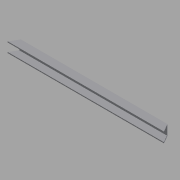
# Autodesk Inventor part: 19in c-channel-top
Saved by Autodesk Inventor 2013 (Build 170138000, 138)
## iProperties
Created: 2013-01-24
Part Number: 19in c-channel-top
Material: Generic
Document SubType Name: Modeling
Designer: Naphat
Density: 1 g/cm^3
Author: Naphat
Autodesk Inventor part; units mm, degrees
ref_plane "YZ Plane" through (0, 0, 0) normal (1, 0, 0) x (0, 1, 0)
ref_plane "XZ Plane" through (0, 0, 0) normal (0, 1, 0) x (-1, 0, 0)
ref_plane "XY Plane" through (0, 0, 0) normal (0, 0, 1) x (1, 0, 0)
sketch "Sketch1" plane through (0, 0, 0) normal (1, 0, 0) x (0, 1, 0)
  line L0 (-15.7, 12.7) -> (-12.7, 12.7)
  line L1 (-12.7, 12.7) -> (-12.7, -9.7)
  line L2 (-12.7, -9.7) -> (12.7, -9.7)
  line L3 (12.7, -9.7) -> (12.7, 12.7)
  line L4 (12.7, 12.7) -> (15.7, 12.7)
  line L5 (15.7, 12.7) -> (15.7, -12.7)
  line L6 (15.7, -12.7) -> (-15.7, -12.7)
  line L7 (-15.7, -12.7) -> (-15.7, 12.7)
  point P0 (0, 0)
  point P1 (0, 0)
  dimension "d0" = 3
  dimension "d1" = 3
  dimension "d2" = 25.4
  dimension "d3" = 31.4
  dimension "d4" = 15.7
  dimension "d5" = 12.7
  dimension "d6" = 3
  constraints: 16 end point, 5 parallel, 1 collinear, 1 horizontal, 1 perpendicular
  measures "d0" distance of L0.start L0.end
  measures "d1" distance of L3.end L4.end
  measures "d2" distance of L6.end L0.start
  measures "d3" distance of L5.end L6.end
  measures "d4" distance from line of point (0, 0) L7
  measures "d5" distance from line of L6 point (0, 0)
  measures "d6" distance between parallel lines of L6 L2
extrude "Extrusion1" add sketch "Sketch1" along normal blind 482.6
sketch "Sketch2" plane through (0, 15.7, 12.7) normal (0, 1, 0) x (1, 0, 0)
  line L0 (482.6, 0) -> (481.8634, 0)
  line L1 (482.6, 25.4) -> (467.2076, 25.4)
  line L2 (467.2076, 25.4) -> (481.8634, 0)
  line L3 (482.6, 0) -> (482.6, 25.4)
  line L4 (0, 0) -> (0.7366, 0)
  line L5 (0, 25.4) -> (15.3924, 25.4)
  line L6 (15.3924, 25.4) -> (0.7366, 0)
  line L7 (0, 25.4) -> (0, 0)
  point P0 (0, 12.7)
  dimension "d9" = 0.7366
  dimension "d10" = 15.3924
  dimension "d11" = 0.7366
  dimension "d12" = 15.3924
  constraints: 16 end point, 1 perpendicular
  measures "d9" distance of L0.start L0.end
  measures "d10" distance of L1.start L1.end
  measures "d11" distance of L4.start L4.end
  measures "d12" distance of L5.start L5.end
extrude "Extrusion2" cut sketch "Sketch2" against normal blind 76.2
equation "\"d1\" = d0"
equation "\"d4\" = 0.5 * d3"
equation "\"d5\" = 0.5 * d2"
equation "\"d6\" = d0"
body "Solid1"
